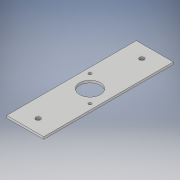
# Autodesk Inventor part: BAGMotor Beam
Saved by Autodesk Inventor 2017 (Build 210142000, 142)
## iProperties
Created: 2016-09-26
Part Number: BAGMotor Beam
Material: Generic
Document SubType Name: Modeling
Designer: Hanson
Density: 1 g/cm^3
Appearance: Default
Author: Hanson
Autodesk Inventor part; units mm, degrees
ref_plane "YZ Plane" through (0, 0, 0) normal (1, 0, 0) x (0, 1, 0)
ref_plane "XZ Plane" through (0, 0, 0) normal (0, 1, 0) x (-1, 0, 0)
sketch "Sketch1" plane through (0, 0, 0) normal (0, 1, 0) x (-1, 0, 0)
  line L0 (0, 0) -> (-25.4, 0)
  line L1 (-25.4, 0) -> (-25.4, -178.054)
  line L2 (-25.4, -178.054) -> (0, -178.054)
  line L3 (0, -178.054) -> (0, 0)
  dimension "d0" = 25.4
  dimension "d1" = 178.054
  constraints: 8 end point, 2 parallel, 1 horizontal, 1 perpendicular
  measures "d0" distance of L2.end L1.end
  measures "d1" distance of L0.end L1.end
extrude "Extrusion1" add sketch "Sketch1" along normal blind 3.175
sketch "Sketch2" plane through (0, 3.175, 0) normal (0, 1, 0) x (1, 0, 0)
  line L0 (0, 178.054) -> (0, 0) projected
  line L1 (0, 0) -> (25.4, 0) projected
  point P0 (12.7, 17.78)
  dimension "d4" = 12.7
  dimension "d5" = 17.78
  measures "d4" distance from line of L0 point (12.7, 17.78)
  measures "d5" distance from line of L1 point (12.7, 17.78)
hole "Hole1" at (12.7, 3.175, -17.78) direction (0, -1, 0) diameter 6.35 end through all
ref_plane "Work Plane1" through (25.4, 0, -89.027) normal (0, 0, -1) x (-1, 0, 0)
mirror "Mirror1" about plane through (25.4, 0, -89.027) normal (0, 0, -1) of "Hole1"
sketch "Sketch3" plane through (25.4, 0, 0) normal (1, 0, 0) x (0, 0, -1)
  line L0 (0, 3.175) -> (178.054, 3.175) projected
  line L1 (0, 0) -> (178.054, 0) projected
  line L2 (0, 3.175) -> (178.054, 3.175)
  line L3 (178.054, 3.175) -> (178.054, 0)
  line L4 (178.054, 0) -> (0, 0)
  line L5 (0, 0) -> (0, 3.175)
  constraints: 8 end point, 2 parallel, 1 horizontal, 1 perpendicular
extrude "Extrusion2" add sketch "Sketch3" along normal blind 12.7
sketch "Sketch4" plane through (0, 0, -178.054) normal (-1, 0, 0) x (0, 0, 1)
  line L0 (0, 0) -> (0, 3.175) projected
  line L1 (178.054, 0) -> (0, 0)
  line L2 (0, 0) -> (0, 3.175)
  line L3 (0, 3.175) -> (178.054, 3.175)
  line L4 (178.054, 3.175) -> (178.054, 0)
  constraints: 8 end point, 2 parallel, 1 horizontal, 1 perpendicular
extrude "Extrusion3" add sketch "Sketch4" along normal blind 12.7
sketch "Sketch5" plane through (0, 3.175, 0) normal (0, 1, 0) x (1, 0, 0)
  line L0 (-12.7, 0) -> (-12.7, 178.054) projected
  line L1 (38.1, 0) -> (-12.7, 0) projected
  point P0 (0, 0)
  point P1 (12.7, 89.027)
  dimension "d17" = 25.4
  dimension "d18" = 89.027
  measures "d17" distance from line of L0 point (12.7, 89.027)
  measures "d18" distance from line of L1 point (12.7, 89.027)
hole "Hole2" at (12.7, 3.175, -89.027) direction (0, -1, 0) diameter 28.5496 end through all
sketch "Sketch6" plane through (0, 3.175, 0) normal (0, 1, 0) x (1, 0, 0)
  line L0 (38.1, 0) -> (-12.7, 0) projected
  line L1 (38.1, 0) -> (38.1, 178.054) projected
  point P0 (0, 0)
  point P1 (30.6578, 71.0692)
  dimension "d26" = 71.0692
  dimension "d27" = 7.4422
  measures "d26" distance from line of L0 point (30.658, 71.069)
  measures "d27" distance from line of L1 point (30.658, 71.069)
hole "Hole3" at (30.6578, 3.175, -71.0692) direction (0, -1, 0) diameter 4.0386 end through all
sketch "Sketch7" plane through (0, 3.175, 0) normal (0, 1, 0) x (1, 0, 0)
  line L0 (-12.7, 0) -> (-12.7, 178.054) projected
  line L1 (-12.7, 178.054) -> (38.1, 178.054) projected
  point P0 (0, 0)
  point P1 (-5.2578, 106.9848)
  dimension "d35" = 7.4422
  dimension "d36" = 71.0692
  measures "d35" distance from line of L0 point (-5.258, 106.985)
  measures "d36" distance from line of L1 point (-5.258, 106.985)
hole "Hole4" at (-5.2578, 3.175, -106.9848) direction (0, -1, 0) diameter 4.0386 end through all
body "Solid1"
